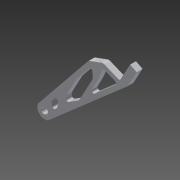
# Autodesk Inventor part: UpperArmGenerative
Saved by Autodesk Inventor 2020 (Build 240168000, 168)
## iProperties
Created: 2020-04-02
Part Number: UpperArmGenerative
Material: Aluminum 6061
Document SubType Name: Modeling
Designer: Administrator
Density: 2.7 g/cm^3
Appearance: White
Title: UpperArmGenerative v7
Author: Administrator
Autodesk Inventor part; units mm, degrees
ref_plane "YZ Plane" through (0, 0, 0) normal (1, 0, 0) x (0, 1, 0)
ref_plane "XZ Plane" through (0, 0, 0) normal (0, 1, 0) x (-1, 0, 0)
ref_plane "XY Plane" through (0, 0, 0) normal (0, 0, 1) x (1, 0, 0)
sketch "Base" plane through (0, 0, 0) normal (0, 0, 1) x (1, 0, 0)
  circle A0 centre (-1.61, 0.369) radius 3.175
  circle A1 centre (-1.61, 0.369) radius 20.32
  circle A2 centre (-330.4664, -297.5763) radius 3.1016
  circle A3 centre (-330.4664, -297.5763) radius 15.875
  line L0 (-312.9479, -300.6623) -> (-300, -300.6623)
  line L1 (-300, -300.6623) -> (-22.6706, -58.9044)
  line L2 (-300, -300.6623) -> (-22.6706, -58.9044)
  line L3 (-22.6706, -58.9044) -> (-1.3645, -19.9495)
  line L4 (-22.6706, -58.9044) -> (-2.3057, -21.6703)
  line L5 (-49.3253, -54.706) -> (-21.4935, -3.8199)
  line L6 (-107.2006, -31.0716) -> (-157.6315, -49.5808)
  line L7 (-49.3253, -54.706) -> (-107.2006, -31.0716)
  line L8 (-107.2006, -31.0716) -> (-157.6315, -49.5808)
  line L9 (-300, -300.6623) -> (-314.8942, -300.6623)
  line L10 (-157.6315, -49.5808) -> (-334.4078, -267.6676)
  line L11 (-103.459, -49.0613) -> (-65.2129, -64.6798)
  line L12 (-64.729, -75.3505) -> (-118.5834, -122.2973)
  line L13 (-136.3823, -111.4893) -> (-127.3923, -94.8521)
  line L14 (-149.2919, -136.0891) -> (-136.3823, -111.4893)
  line L15 (-56.5476, -68.2184) -> (-107.4943, -47.4135)
  line L16 (-56.5476, -68.2184) -> (-161.8454, -160.0103)
  line L17 (-142.5707, -96.2269) -> (-162.074, -132.3201)
  line L18 (-198.9013, -124.6971) -> (-233.9187, -189.5013)
  line L19 (-161.8454, -160.0103) -> (-136.3823, -111.4893)
  line L20 (-127.3923, -94.8521) -> (-136.3823, -111.4893)
  line L21 (-198.9013, -124.6971) -> (-145.6271, -58.9735)
  line L22 (-190.565, -185.0462) -> (-142.5707, -96.2269)
  line L23 (-142.5707, -96.2269) -> (-145.6271, -58.9735)
  line L24 (-314.8942, -288.0888) -> (-322.3347, -280.1945)
  line L25 (-314.8942, -288.0888) -> (-322.3347, -280.1945)
  line L26 (-322.3347, -280.1945) -> (-317.4135, -269.9997)
  line L27 (-322.3347, -280.1945) -> (-317.4135, -269.9997)
  line L28 (-304.4264, -283.7813) -> (-314.8942, -288.0888)
  arc A4 (-304.4264, -283.7813) -> (-317.4135, -269.9997) centre (-308.2841, -274.4066) ccw
  line L29 (-304.4264, -283.7813) -> (-314.8942, -288.0888)
  line L30 (-161.8454, -160.0103) -> (-190.565, -185.0462) construction
  line L31 (-190.565, -185.0462) -> (-237.1335, -214.697)
  line L32 (-237.1335, -214.697) -> (-233.9187, -189.5013)
  line L33 (-21.4935, -3.8199) -> (-13.3975, 10.9824)
  line L34 (-13.3975, 10.9824) -> (9.3449, -0.369)
  line L35 (9.3449, -0.369) -> (-1.5358, -20.2627)
  line L36 (-334.4078, -282.1983) -> (-334.4078, -267.6676)
  line L37 (-314.8942, -300.6623) -> (-320.7087, -300.6623)
  line L38 (-320.7087, -300.6623) -> (-334.4078, -285.9351)
  line L39 (-334.4078, -285.9351) -> (-334.4078, -282.1983)
  line L40 (-284.0273, -244.2885) -> (-286.1104, -229.4747) construction
  line L41 (-261.2714, -210.7778) -> (-286.1104, -230.099)
  line L42 (-265.5633, -244.4149) -> (-281.6579, -261.2388)
  line L43 (-265.5633, -244.4149) -> (-261.2714, -210.7778)
  line L44 (-281.6579, -261.2388) -> (-286.044, -230.0474)
  line L45 (-107.4943, -47.4135) -> (-127.3923, -94.8521)
  point P0 (0, 0)
  point P1 (0, 0)
  point P2 (-2.3057, -21.6703)
  point P3 (-1.3645, -19.9495)
  point P4 (-213.8492, -199.8716)
  dimension "d3" = 40.64
  dimension "d4" = 31.75
  dimension "d7" = 15.24
  dimension "d8" = 15.24
  dimension "d11" = 12.7
  dimension "d12" = 38.1
  dimension "d13" = 15.24
  dimension "d16" = 8.594
  dimension "d17" = 10.643
  dimension "d18" = 73.66
  dimension "d19" = 25.4
  dimension "d137" = 43.718
  dimension "d138" = 84.6034
  dimension "d140" = 15.24
  constraints: 95 end point, 15 collinear, 7 parallel, 6 point on circle, 6 point on line, 5 centre point, 3 tangent, 2 coincident, 1 horizontal, 1 midpoint, 1 perpendicular, 1 vertical, 7 other
  measures "d3" diameter of A1
  measures "d4" diameter of A3
  measures "d7" distance between parallel lines of L1 L16
  measures "d8" distance between parallel lines of L7 L11
  measures "d11" distance between parallel lines of L13 L17
  measures "d12" distance of L22.start L16.end
  measures "d13" distance between parallel lines of L10 L21
  measures "d16" angle of L1 L31
  measures "d17" angle of L10 L18
  measures "d18" distance of L18.start L18.end
  measures "d19" distance of L31.end L18.end
  measures "d137" angle of L23 L21
  measures "d138" distance of L18.start L21.end
  measures "d140" distance from line of L6 L15.end
extrude "BaseFeature" add sketch "Base" along normal blind 20.32 contours A0 | L33 L34 L35 A1 | A1 L3 L1 L0 L9 A3 L36 L10 L6 L7 L5 | A3 L37 L38 L39 picked at (-13.2253, 2.5105) picked at (-325.2834, -290.544)
fillet "InsideFilletsFeature" radius 6.35 16 edges at (-314.8942, -288.0888, 10.16) (-322.3347, -280.1945, 10.16) (-190.565, -185.0462, 10.16) (-237.1335, -214.697, 10.16) (-142.5707, -96.2269, 10.16) (-56.5476, -68.2184, 10.16) (-161.8454, -160.0103, 10.16) (-49.3253, -54.706, 10.16) (-265.5633, -244.4149, 10.16) (-286.044, -230.0474, 10.16) (-261.2714, -210.7778, 10.16) (-281.6579, -261.2388, 10.16) (-233.9187, -189.5013, 10.16) (-198.9013, -124.6971, 10.16) (-145.6271, -58.9735, 10.16) (-107.4943, -47.4135, 10.16)
fillet "InsideFilletLargeFeature" radius 25.4 1 edges at (-127.3923, -94.8521, 10.16)
fillet "OutsideFilletsFeature" radius 12.7 7 edges at (-107.2006, -31.0716, 10.16) (-157.6315, -49.5808, 10.16) (-22.6706, -58.9044, 10.16) (-300, -300.6623, 10.16) (-320.7087, -300.6623, 10.16) (-334.4078, -285.9351, 10.16) (-334.4078, -267.6676, 10.16)
sketch "Sketch3" plane through (0, 0, 20.32) normal (0, 0, 1) x (1, 0, 0)
  line L0 (-64.3139, -74.9886) -> (-136.3059, -137.7466) projected
  line L1 (-191.9567, -185.9323) -> (-225.7101, -207.4235) construction
  arc A0 (-283.1429, -227.7907) -> (-285.5322, -233.6871) centre (-279.2441, -232.8029) ccw projected
  line L2 (-267.009, -245.9262) -> (-272.6049, -251.7756) projected
  line L3 (-198.1564, -123.7782) -> (-283.1429, -227.7907)
  arc A1 (-267.009, -245.9262) -> (-265.2986, -242.3403) centre (-271.5975, -241.5366) ccw projected
  arc A2 (-304.4264, -283.7813) -> (-317.4135, -269.9997) centre (-308.2841, -274.4066) ccw projected
  line L4 (-283.1429, -227.7907) -> (-316.1205, -267.9757)
  line L5 (-103.8082, -48.9187) -> (-107.4943, -47.4135)
  line L6 (-107.4943, -47.4135) -> (-148.4373, -62.4404)
  line L7 (-148.4373, -62.4404) -> (-155.5945, -71.2701)
  line L8 (-101.6709, -49.7915) -> (-66.0859, -64.3233) projected
  line L9 (-111.8211, -32.7675) -> (-154.3454, -48.3748) projected
  arc A3 (-64.3139, -74.9886) -> (-66.0859, -64.3233) centre (-68.4866, -70.202) ccw projected
  line L10 (-320.4349, -276.2589) -> (-317.4135, -269.9997) projected
  arc A4 (-320.4349, -276.2589) -> (-319.3373, -283.3747) centre (-314.7163, -279.0194) ccw projected
  line L11 (-317.8911, -284.9092) -> (-319.3373, -283.3747) projected
  arc A5 (-317.8911, -284.9092) -> (-310.8536, -286.4261) centre (-313.2701, -280.5539) ccw projected
  line L12 (-304.4264, -283.7813) -> (-310.8536, -286.4261) projected
  arc A6 (-304.4264, -283.7813) -> (-317.4135, -269.9997) centre (-308.2841, -274.4066) ccw projected
  line L13 (-136.3059, -137.7466) -> (-301.6178, -282.0438)
  line L14 (-198.5288, -124.2377) -> (-155.5945, -71.2701) projected
  point P0 (0, 0)
  point P1 (-284.9207, -229.9571)
  dimension "d27" = 15.24
  constraints: 12 end point, 3 tangent, 2 point on circle, 1 collinear, 1 parallel
  measures "d27" distance between parallel lines of L9 L6
extrude "Extrusion2" [suppressed]
sketch "Sketch4" plane through (0, 0, 20.32) normal (0, 0, 1) x (1, 0, 0)
  line L0 (-283.1429, -227.7907) -> (-198.1564, -123.7782) projected
  arc A0 (-253.1902, -219.8511) -> (-235.4994, -224.3305) centre (-242.8218, -216.0758) ccw
  arc A1 (-253.1902, -219.8511) -> (-261.9051, -201.7984) centre (-286.1514, -224.6332) ccw
  arc A2 (-283.1429, -227.7907) -> (-284.9207, -229.9571) centre (-279.2441, -232.8029) ccw projected
  line L1 (-316.1205, -267.9757) -> (-284.9207, -229.9571) projected
  arc A3 (-316.1205, -267.9757) -> (-317.4135, -269.9997) centre (-308.2841, -274.4066) ccw projected
  arc A4 (-316.1205, -267.9757) -> (-317.4135, -269.9997) centre (-308.2841, -274.4066) ccw projected
  line L2 (-304.4264, -283.7813) -> (-310.8536, -286.4261) projected
  arc A5 (-317.8911, -284.9092) -> (-310.8536, -286.4261) centre (-313.2701, -280.5539) ccw projected
  line L3 (-317.8911, -284.9092) -> (-319.3373, -283.3747) projected
  arc A6 (-320.4349, -276.2589) -> (-319.3373, -283.3747) centre (-314.7163, -279.0194) ccw projected
  line L4 (-320.4349, -276.2589) -> (-317.4135, -269.9997) projected
  line L5 (-265.2986, -242.3403) -> (-263.2189, -226.0409) projected
  arc A7 (-267.009, -245.9262) -> (-265.2986, -242.3403) centre (-271.5975, -241.5366) ccw projected
  line L6 (-272.6049, -251.7756) -> (-267.009, -245.9262) projected
  arc A8 (-283.4815, -248.2703) -> (-272.6049, -251.7756) centre (-277.1934, -247.3861) ccw projected
  line L7 (-285.5322, -233.6871) -> (-283.4815, -248.2703) projected
  arc A9 (-284.9207, -229.9571) -> (-285.5322, -233.6871) centre (-279.2441, -232.8029) ccw projected
  arc A10 (-283.1429, -227.7907) -> (-285.5322, -233.6871) centre (-279.2441, -232.8029) ccw projected
  line L8 (-273.4166, -220.225) -> (-283.1429, -227.7907) projected
  arc A11 (-263.2189, -226.0409) -> (-273.4166, -220.225) centre (-269.5178, -225.2372) ccw projected
  arc A12 (-301.6178, -282.0438) -> (-316.1205, -267.9757) centre (-308.2841, -274.4066) ccw projected
  line L9 (-136.3059, -137.7466) -> (-301.6178, -282.0438) projected
  point P0 (0, 0)
  point P1 (-235.6322, -224.4465)
  constraints: 4 point on circle, 2 centre point, 2 point on line
sketch "Sketch6" plane through (0, 0, 0) normal (0, 0, -1) x (-1, 0, 0)
  arc A0 (317.4135, -269.9997) -> (304.4264, -283.7813) centre (308.2841, -274.4066) ccw projected
  arc A1 (272.6049, -251.7756) -> (283.4815, -248.2703) centre (277.1934, -247.3861) ccw projected
  line L0 (283.4815, -248.2703) -> (285.5322, -233.6871) projected
  arc A2 (285.5322, -233.6871) -> (283.1429, -227.7907) centre (279.2441, -232.8029) ccw projected
  line L1 (300.9589, -281.4143) -> (272.6049, -251.7756)
  line L2 (316.1404, -268) -> (284.1652, -228.7898)
  point P0 (0, 0)
  constraints: 4 end point, 3 point on circle, 3 tangent
sketch "Sketch7" plane through (-296.4131, -297.5355, -7.62) normal (0.6571099, -0.7537948, 0) x (0.7537948, 0.6571099, 0)
  line L0 (-8.3453, 0) -> (-8.3453, 15.24)
  line L1 (0, 15.24) -> (-8.3453, 15.24)
  line L2 (0, 0) -> (-8.3453, 0)
  line L3 (0, 15.24) -> (55.1547, 15.24)
  line L4 (55.1547, 15.24) -> (55.1547, 0)
  line L5 (55.1547, 0) -> (-4.1726, 0)
  line L6 (0, 0) -> (360.8853, 0) projected
  line L7 (0, 15.24) -> (360.8853, 15.24) projected
  point P0 (418.9482, 7.62)
  point P1 (-8.3453, 15.24)
  dimension "d59" = 63.5
  constraints: 12 end point, 2 collinear, 1 midpoint
  measures "d59" distance between parallel lines of L0 L4
sketch "Sketch9" plane through (-331.5738, -264.1713, -7.62) normal (-0.7768442, 0.6296929, 0) x (0, 0, 1)
  line L0 (0, 0) -> (15.24, 0)
  line L1 (15.24, 0) -> (15.24, 50.8)
  line L2 (15.24, 50.8) -> (0, 50.8)
  line L3 (0, 50.8) -> (0, 0)
  line L4 (15.24, 272.7332) -> (15.24, 0) projected
  line L5 (0, 272.7332) -> (0, 0) projected
  line L6 (15.24, 0) -> (0, 0) projected
  point P0 (7.62, 414.0095)
  point P1 (15.24, 201.6132)
  point P2 (0, 201.6132)
  dimension "d71" = 0
  dimension "d72" = 50.8
  dimension "d89" = 50.8
  constraints: 8 end point, 2 coincident, 2 parallel, 1 centre point, 1 horizontal, 1 midpoint, 1 perpendicular, 5 other
sketch "Sketch12" plane through (0, 0, 20.32) normal (0, 0, 1) x (1, 0, 0)
  circle A0 centre (-249.2375, -200.025) radius 3.175
  circle A1 centre (-242.8218, -216.0758) radius 3.175
  point P0 (0, 0)
  dimension "d107" = 6.35
  constraints: 2 centre point, 1 coincident, 1 equal radius, 1 other
  measures "d107" diameter of A0
sketch "Sketch13" plane through (-159.8356, -52.3001, -7.62) normal (-0.7768442, 0.6296929, 0) x (0, 0, 1)
  line L0 (-2.54, -10.2019) -> (17.78, -10.2019)
  line L1 (17.78, -10.2019) -> (17.78, 41.8025)
  line L2 (17.78, 41.8025) -> (-2.54, 41.8025)
  line L3 (-2.54, 41.8025) -> (-2.54, -10.2019)
  line L4 (7.62, 26.3292) -> (7.62, 39.3729) projected
  point P0 (7.62, 141.2763)
  point P1 (7.62, 41.8025)
  dimension "d112" = 20.32
  constraints: 8 end point, 2 parallel, 1 horizontal, 1 midpoint, 1 perpendicular, 1 point on line
  measures "d112" distance of L0.start L0.end
sketch "Sketch17" plane through (-111.8211, -32.7675, 7.62) normal (-0.3445481, 0.9387687, 0) x (0.9387687, 0.3445481, 0)
  ellipse E0 centre (-30.8051, 7.5999) end of major axis (-30.8051, -7.6401) minor radius 14.7541 (-26.4891, 22.1732) -> (-26.3638, -6.9332) ccw construction
  line L0 (-26.3638, -6.9332) -> (-10.702, -1.905) construction
  line L1 (-26.2826, -7.1841) -> (-10.4383, -2.0973)
  line L2 (-10.4383, -2.0973) -> (-10.4383, 17.3377)
  line L3 (-10.4383, 17.3377) -> (-26.4094, 22.4246)
  spline S0 degree 5 poles (-26.4094, 22.4245) (-27.5905, 22.7978) (-28.811, 23.0464) (-30.0535, 23.1639) (-34.273, 23.1093) (-38.3151, 21.5552) (-40.8163, 19.7483) (-44.7675, 15.0619) (-46.1888, 9.0911) (-46.1756, 5.9687) (-44.7032, 0.0107) (-40.7111, -4.6402) (-38.194, -6.4241) (-34.1386, -7.9408) (-29.9195, -7.9566) (-28.6783, -7.8277) (-27.4602, -7.568) (-26.2826, -7.184) knots 0 0 0 0 0 0 0.10864 0.10864 0.10864 0.368033 0.368033 0.368033 0.632034 0.632034 0.632034 0.89137 0.89137 0.89137 1 1 1 1 1 1
  point P0 (116.2641, 7.62)
  constraints: 6 end point, 7 other
body "Solid2"
